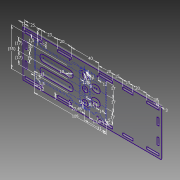
# Autodesk Inventor part: Bottom_plate2
Saved by Autodesk Inventor 2015 (Build 190159000, 159)
## iProperties
Created: 2015-06-18
Part Number: Bottom_plate2
Material: Generic
Document SubType Name: Modeling
Designer: Openlab
Density: 1 g/cm^3
Appearance: Polycarbonate - Clear
Author: Openlab
Autodesk Inventor part; units mm, degrees
ref_plane "YZ Plane" through (0, 0, 0) normal (1, 0, 0) x (0, 1, 0)
ref_plane "XZ Plane" through (0, 0, 0) normal (0, 1, 0) x (-1, 0, 0)
ref_plane "XY Plane" through (0, 0, 0) normal (0, 0, 1) x (1, 0, 0)
sketch "Sketch1" plane through (0, 0, 0) normal (0, 1, 0) x (-1, 0, 0)
  line L0 (37.25, -2.25) -> (24.75, -2.25) construction
  line L1 (24.75, -2.25) -> (24.75, -14.75) construction
  line L2 (24.75, -14.75) -> (37.25, -14.75) construction
  line L3 (37.25, -14.75) -> (37.25, -2.25) construction
  line L4 (56.9183, -8.5) -> (8.3915, -8.5) construction
  line L5 (0, -17) -> (105, -17) construction
  line L6 (0, 0) -> (0, -51) construction
  line L7 (0, -34) -> (105, -34) construction
  line L8 (105, -51) -> (105, 0) construction
  line L9 (31, 5) -> (31, -51) construction
  line L10 (56.8064, -25.5) -> (17, -25.5) construction
  line L11 (24.75, -19.25) -> (24.75, -31.75) construction
  line L12 (37.25, -19.25) -> (24.75, -19.25) construction
  line L13 (37.25, -31.75) -> (37.25, -19.25) construction
  line L14 (24.75, -31.75) -> (37.25, -31.75) construction
  line L15 (24.75, -36.25) -> (24.75, -48.75) construction
  line L16 (37.25, -36.25) -> (24.75, -36.25) construction
  line L17 (37.25, -48.75) -> (37.25, -36.25) construction
  line L18 (24.75, -48.75) -> (37.25, -48.75) construction
  line L19 (56.3008, -42.5) -> (16.5498, -42.5) construction
  arc A0 (53.45, -12) -> (53.45, -22) centre (53.45, -17) ccw
  arc A1 (92, -22) -> (92, -12) centre (92, -17) ccw
  arc A2 (53.45, -29) -> (53.45, -39) centre (53.45, -34) ccw
  arc A3 (92, -39) -> (92, -29) centre (92, -34) ccw
  line L20 (53.45, -12) -> (92, -12)
  line L21 (53.45, -22) -> (92, -22)
  line L22 (53.45, -29) -> (92, -29)
  line L23 (53.45, -39) -> (92, -39)
  arc A4 (16.65, -39) -> (16.65, -29) centre (16.65, -34) ccw
  line L24 (103.5, -49.5) -> (103.5, -1.5) construction
  line L25 (1.5, -1.5) -> (1.5, -49.5) construction
  arc A5 (14, -29) -> (14, -39) centre (14, -34) ccw
  arc A6 (14, -12) -> (14, -22) centre (14, -17) ccw
  line L26 (16.65, -39) -> (14, -39)
  line L27 (14, -29) -> (16.65, -29)
  line L28 (14, -22) -> (16.65, -22)
  line L29 (16.65, -12) -> (14, -12)
  arc A7 (16.65, -22) -> (16.65, -12) centre (16.65, -17) ccw
  arc A8 (96.5, -51) -> (93, -47.5) centre (93, -51) ccw construction
  arc A9 (53.45, -47.5) -> (49.95, -51) centre (53.45, -51) ccw construction
  arc A10 (97.7697, -49.5) -> (93, -46) centre (93, -51) ccw construction
  line L30 (93, -46) -> (53.45, -46) construction
  line L31 (96.5, -51) -> (105, -51) construction
  line L32 (93, -47.5) -> (53.45, -47.5) construction
  line L33 (105, -49.5) -> (97.7697, -49.5) construction
  arc A11 (53.45, -46) -> (48.6803, -49.5) centre (53.45, -51) ccw construction
  arc A12 (48.6803, -1.5) -> (53.45, -5) centre (53.45, 0) ccw construction
  arc A13 (49.95, 0) -> (53.45, -3.5) centre (53.45, 0) ccw construction
  line L34 (93, -3.5) -> (53.45, -3.5) construction
  line L35 (93, -5) -> (53.45, -5) construction
  line L36 (97.7697, -1.5) -> (105, -1.5) construction
  line L37 (105, 0) -> (96.5, 0) construction
  arc A14 (93, -3.5) -> (96.5, 0) centre (93, 0) ccw construction
  arc A15 (93, -5) -> (97.7697, -1.5) centre (93, 0) ccw construction
  arc A16 (16.65, -51) -> (13.15, -47.5) centre (13.15, -51) ccw construction
  arc A17 (12, -47.5) -> (8.5, -51) centre (12, -51) ccw construction
  line L38 (13.15, -46) -> (12, -46) construction
  line L39 (13.15, -47.5) -> (12, -47.5) construction
  arc A18 (12, -46) -> (7.2303, -49.5) centre (12, -51) ccw construction
  arc A19 (17.9197, -49.5) -> (13.15, -46) centre (13.15, -51) ccw construction
  line L40 (48.6803, -49.5) -> (17.9197, -49.5) construction
  line L41 (7.2303, -49.5) -> (0, -49.5) construction
  line L42 (0, -51) -> (8.5, -51) construction
  line L43 (16.65, -51) -> (49.95, -51) construction
  line L44 (13.15, -5) -> (12, -5) construction
  line L45 (13.15, -3.5) -> (12, -3.5) construction
  arc A20 (8.5, 0) -> (12, -3.5) centre (12, 0) ccw construction
  arc A21 (13.15, -3.5) -> (16.65, 0) centre (13.15, 0) ccw construction
  arc A22 (7.2303, -1.5) -> (12, -5) centre (12, 0) ccw construction
  arc A23 (13.15, -5) -> (17.9197, -1.5) centre (13.15, 0) ccw construction
  line L46 (49.95, 0) -> (16.65, 0) construction
  line L47 (8.5, 0) -> (0, 0) construction
  line L48 (0, -1.5) -> (7.2303, -1.5) construction
  line L49 (17.9197, -1.5) -> (48.6803, -1.5) construction
  arc A24 (38.75, -4.25) -> (35.25, -0.75) centre (35.25, -4.25) ccw construction
  arc A25 (26.75, -0.75) -> (23.25, -4.25) centre (26.75, -4.25) ccw construction
  arc A26 (35.25, -50.25) -> (38.75, -46.75) centre (35.25, -46.75) ccw construction
  arc A27 (23.25, -46.75) -> (26.75, -50.25) centre (26.75, -46.75) ccw construction
  line L50 (38.75, -4.25) -> (38.75, -46.75) construction
  line L51 (35.25, -0.75) -> (26.75, -0.75) construction
  line L52 (23.25, -4.25) -> (23.25, -46.75) construction
  line L53 (26.75, -50.25) -> (35.25, -50.25) construction
  line L54 (119, 2) -> (119, 5)
  line L55 (-77, 5) -> (-77, 2)
  line L56 (119, -53) -> (119, -56)
  line L57 (122, 8) -> (122, -59)
  line L58 (-80, -59) -> (-80, 8)
  line L59 (51, 5) -> (51, 2)
  line L60 (71, 5) -> (71, 2)
  line L61 (94, 5) -> (94, 2)
  line L62 (11, 5) -> (11, 2)
  line L63 (-9, 2) -> (-9, 5)
  line L64 (51, -56) -> (51, -53)
  line L65 (11, -56) -> (11, -53)
  line L66 (-9, -56) -> (-9, -53)
  line L67 (71, -56) -> (71, -53)
  line L68 (94, -56) -> (94, -53)
  line L69 (-24, 5) -> (-24, 2)
  line L70 (-24, -53) -> (-24, -56)
  line L71 (122, 8) -> (-80, 8)
  line L72 (-80, -59) -> (122, -59)
  line L73 (11, 5) -> (-9, 5)
  line L74 (11, 2) -> (-9, 2)
  line L75 (119, 5) -> (94, 5)
  line L76 (71, 5) -> (51, 5)
  line L77 (119, 2) -> (94, 2)
  line L78 (71, 2) -> (51, 2)
  line L79 (51, -53) -> (71, -53)
  line L80 (94, -53) -> (119, -53)
  line L81 (119, -56) -> (94, -56)
  line L82 (71, -56) -> (51, -56)
  line L83 (-9, -53) -> (11, -53)
  line L84 (11, -56) -> (-9, -56)
  line L85 (-39, 5) -> (-39, 2)
  line L86 (-59, 5) -> (-59, 2)
  line L87 (-39, -53) -> (-39, -56)
  line L88 (-59, -53) -> (-59, -56)
  line L89 (-24, 5) -> (-39, 5)
  line L90 (-59, 5) -> (-77, 5)
  line L91 (-24, 2) -> (-39, 2)
  line L92 (-59, 2) -> (-77, 2)
  line L93 (-77, -53) -> (-59, -53)
  line L94 (-39, -53) -> (-24, -53)
  line L95 (-24, -56) -> (-39, -56)
  line L96 (-59, -56) -> (-77, -56)
  line L97 (119, -8) -> (116, -8)
  line L98 (116, -8) -> (116, -18)
  line L99 (116, -18) -> (119, -18)
  line L100 (119, -18) -> (119, -8)
  line L101 (-77, -56) -> (-77, -53)
  line L102 (119, -33) -> (116, -33)
  line L103 (116, -33) -> (116, -43)
  line L104 (116, -43) -> (119, -43)
  line L105 (119, -43) -> (119, -33)
  line L106 (-74, -8) -> (-77, -8)
  line L107 (-77, -8) -> (-77, -18)
  line L108 (-77, -18) -> (-74, -18)
  line L109 (-74, -18) -> (-74, -8)
  line L110 (-74, -33) -> (-77, -33)
  line L111 (-77, -33) -> (-77, -43)
  line L112 (-77, -43) -> (-74, -43)
  line L113 (-74, -43) -> (-74, -33)
  circle A28 centre (31, -8.5) radius 4
  circle A29 centre (31, -25.5) radius 4
  circle A30 centre (31, -42.5) radius 4
  dimension "d0" = 12.5
  dimension "d1" = 12.5
  dimension "d2" = 17
  dimension "d3" = 31
  dimension "d4" = 105
  dimension "d5" = 17
  dimension "d6" = 17
  dimension "d7" = 10
  dimension "d8" = 1.5
  dimension "d9" = 1.5
  dimension "d10" = 5
  dimension "d11" = 1.5
  dimension "d12" = 1.5
  dimension "d13" = 1.5
  dimension "d14" = 17
  dimension "d15" = 17
  dimension "d16" = 12
  dimension "d17" = 13
  dimension "d19" = 11.6
  dimension "d21" = 12
  dimension "d28" = 2
  dimension "d29" = 2
  dimension "d30" = 7
  dimension "d31" = 2
  dimension "d32" = 2
  dimension "d44" = 40
  dimension "d45" = 20
  dimension "d46" = 15
  dimension "d47" = 20
  dimension "d48" = 23
  dimension "d51" = 3
  dimension "d52" = 2
  dimension "d55" = 14
  dimension "d56" = 8.1
  dimension "d57" = 22.45
  dimension "d58" = 15
  dimension "d59" = 20
  dimension "d60" = 18
  dimension "d66" = 3
  dimension "d67" = 3
  dimension "d69" = 3
  dimension "d70" = 25
  dimension "d71" = 10
  dimension "d73" = 15
  dimension "d74" = 55
  dimension "d75" = 8
  constraints: 228 end point, 86 perpendicular, 56 point on circle, 41 collinear, 41 parallel, 32 point on line, 32 tangent, 31 centre point, 26 equal radius, 19 horizontal, 13 coincident, 12 vertical alignment, 9 horizontal alignment, 8 equal length, 3 vertical, 12 other
  measures "d0" distance of L2.end L1.end
  measures "d1" distance of L0.end L1.end
  measures "d2" distance between parallel lines of L10 L4
  measures "d3" distance between parallel lines of L6 L9
  measures "d4" distance between parallel lines of L6 L8
  measures "d5" distance between parallel lines of L19 L10
  measures "d6" distance between parallel lines of L5 L7
  measures "d7" diameter of A0
  measures "d8" distance between parallel lines of L6 L25
  measures "d9" distance between parallel lines of L8 L24
  measures "d10" radius of A4
  measures "d11" radial gap between concentric circles of A8 A10
  measures "d12" distance between parallel lines of L37 L36
  measures "d13" distance between parallel lines of L41 L42
  measures "d14" distance between parallel lines of L7 L42
  measures "d15" distance between parallel lines of L47 L5
  measures "d16" distance from line of A8.centre L8
  measures "d17" distance from line of L8 A3.centre
  measures "d19" distance from line of A19.centre L15
  measures "d21" distance from line of L6 A22.centre
  measures "d28" distance from line of L1 A25.centre
  measures "d29" distance from line of A25.centre L0
  measures "d30" diameter of A25
  measures "d31" distance from line of L17 A26.centre
  measures "d32" distance from line of L18 A26.centre
  measures "d44" distance between parallel lines of L62 L59
  measures "d45" distance between parallel lines of L63 L62
  measures "d46" distance between parallel lines of L69 L63
  measures "d47" distance between parallel lines of L60 L59
  measures "d48" distance between parallel lines of L61 L60
  measures "d51" distance between parallel lines of L82 L79
  measures "d52" distance between parallel lines of L77 L37
  measures "d55" distance from line of L6 A5.centre
  measures "d56" distance from line of L15 A4.centre
  measures "d57" distance from line of L9 A9.centre
  measures "d58" distance between parallel lines of L85 L69
  measures "d59" distance between parallel lines of L85 L86
  measures "d60" distance between parallel lines of L55 L86
  measures "d66" distance between parallel lines of L71 L75
  measures "d67" distance between parallel lines of L58 L55
  measures "d69" distance between parallel lines of L57 L54
  measures "d70" distance of L54.end L61.start
  measures "d71" distance of L97.end L98.end
  measures "d73" distance between parallel lines of L102 L99
  measures "d74" distance between parallel lines of L80 L77
  measures "d75" diameter of A28
extrude "Extrusion2" add sketch "Sketch1" along normal blind 3
body "Solid1"
